Autodesk Fusion 360 part; units mm, degrees
(part 2 of 2)
sketch "Sketch23" plane through (0, 5, 0) normal (0, 1, 0) x (-1, 0, 0)
  circle A0 centre (-181.5, -92.25) radius 5
  circle A1 centre (-181.5, -115.25) radius 5
  circle A2 centre (-154.5, -126.75) radius 5
  circle A3 centre (-154.5, -103.75) radius 5
  circle A4 centre (-186.75, -72.25) radius 4
  circle A5 centre (-140.75, -72.25) radius 4
  circle A6 centre (-94.75, -72.25) radius 4
  circle A7 centre (-48.75, -72.25) radius 4
  circle A8 centre (-190, -170) radius 3.75
  circle A9 centre (-13.25, -72.25) radius 4
  circle A10 centre (-59.25, -72.25) radius 4
  circle A11 centre (-105.25, -72.25) radius 4
  circle A12 centre (-151.25, -72.25) radius 4
  circle A13 centre (-154.5, -92.25) radius 5
  circle A14 centre (-154.5, -115.25) radius 5
  circle A15 centre (-181.5, -126.75) radius 5
  circle A16 centre (-181.5, -103.75) radius 5
  line L0 (-116.5, -98) -> (-126.5, -98)
  line L1 (-126.5, -98) -> (-126.5, -88)
  line L2 (-126.5, -88) -> (-116.5, -88)
  line L3 (-116.5, -88) -> (-116.5, -98)
  line L4 (0, -101) -> (-8, -101)
  line L5 (-8, -101) -> (-8, -85)
  line L6 (-8, -85) -> (0, -85)
  line L7 (0, -85) -> (0, -67)
  line L8 (0, -67) -> (-8, -67)
  line L9 (-8, -67) -> (-8, -51)
  line L10 (-8, -51) -> (0, -51)
  line L11 (0, -51) -> (0, -11)
  line L12 (0, -11) -> (-6.3858, -11)
  arc A17 (-12.9938, -7.7418) -> (-6.3858, -11) centre (-10, -10) ccw
  arc A18 (-14.6419, 0) -> (-12.9938, -7.7418) centre (-13.25, -3.75) ccw
  line L13 (-14.6419, 0) -> (-47.3581, 0)
  arc A19 (-50.1419, 0) -> (-47.3581, 0) centre (-48.75, -3.75) ccw
  line L14 (-50.1419, 0) -> (-57.8581, 0)
  arc A20 (-60.6419, 0) -> (-57.8581, 0) centre (-59.25, -3.75) ccw
  line L15 (-60.6419, 0) -> (-93.3581, 0)
  arc A21 (-96.1419, 0) -> (-93.3581, 0) centre (-94.75, -3.75) ccw
  line L16 (-96.1419, 0) -> (-103.8581, 0)
  arc A22 (-106.6419, 0) -> (-103.8581, 0) centre (-105.25, -3.75) ccw
  line L17 (-106.6419, 0) -> (-139.3581, 0)
  arc A23 (-142.1419, 0) -> (-139.3581, 0) centre (-140.75, -3.75) ccw
  line L18 (-142.1419, 0) -> (-149.8581, 0)
  arc A24 (-152.6419, 0) -> (-149.8581, 0) centre (-151.25, -3.75) ccw
  line L19 (-152.6419, 0) -> (-185.3581, 0)
  arc A25 (-187.0062, -7.7418) -> (-185.3581, 0) centre (-186.75, -3.75) ccw
  arc A26 (-193.6142, -11) -> (-187.0062, -7.7418) centre (-190, -10) ccw
  line L20 (-193.6142, -11) -> (-200, -11)
  line L21 (-200, -11) -> (-200, -65)
  line L22 (-200, -65) -> (-192, -65)
  line L23 (-192, -65) -> (-192, -78)
  line L24 (-192, -78) -> (-200, -78)
  line L25 (-200, -78) -> (-200, -180)
  line L26 (-200, -180) -> (-180, -180)
  line L27 (-180, -180) -> (-180, -140)
  line L28 (-180, -140) -> (-124.5, -140)
  line L29 (-124.5, -140) -> (-124.5, -110)
  line L30 (-124.5, -110) -> (-55.5, -110)
  line L31 (-55.5, -110) -> (-55.5, -140)
  line L32 (-55.5, -140) -> (-8, -140)
  line L33 (-8, -140) -> (-8, -129)
  line L34 (-8, -129) -> (0, -129)
  line L35 (0, -129) -> (0, -101)
  line L36 (-55.5, -110) -> (-124.5, -110)
  line L37 (-124.5, -110) -> (-124.5, -115)
  line L38 (-124.5, -115) -> (-55.5, -115)
  line L39 (-55.5, -115) -> (-55.5, -110)
  dimension "d326" = 69
  dimension "d327" = 5
  constraint horizontal L36
  constraint vertical L37
  constraint horizontal L38
  constraint vertical L39
  constraint coincident L30.end L31.start
  measures "d326" distance of L30.end L29.end
  measures "d327" distance of L30.end L38.end
extrude "Extrude18" add sketch "Sketch23" along normal blind 11.5 separate body contours L29 L30 L31 L36 L37 L38 L39 makes body 3
combine "Combine1" operation cut target body 3 tool bodies 1 keep tools
sketch "Sketch24" plane through (0, 16.5, 0) normal (0, 1, 0) x (-1, 0, 0)
  line L0 (-119.5, -110) -> (-119.5, -115)
  line L1 (-119.5, -115) -> (-60.5, -115)
  line L2 (-60.5, -115) -> (-60.5, -110)
  line L3 (-60.5, -110) -> (-119.5, -110)
  line L4 (-119.5, -115) -> (-115.5, -115)
  line L5 (-115.5, -115) -> (-115.5, -119)
  line L6 (-115.5, -119) -> (-119.5, -119)
  line L7 (-119.5, -119) -> (-119.5, -115)
  dimension "d330" = 4
  dimension "d331" = 4
  constraint horizontal L4
  constraint vertical L5
  constraint horizontal L6
  constraint vertical L7
  constraint coincident L0.end L1.start
  measures "d330" distance of L0.end L4.end
  measures "d331" distance of L0.end L6.end
extrude "Extrude19" add sketch "Sketch24" against normal blind 5 contours L1 L4 L5 L6 L7 bodies 3
hole "Hole35" at (78.25, 10, -112.5) direction (0, -1, 0) diameter 2.5 end through all bodies 1
hole "Hole36" at (101.75, 10, -112.5) direction (0, -1, 0) diameter 2.5 end through all bodies 1
sketch "Sketch26" plane through (0, 10, 0) normal (0, 1, 0) x (-1, 0, 0)
  circle A0 centre (-78.25, -112.5) radius 1.25
  line L0 (-68.5, -115) -> (-68.5, -110)
  line L1 (-68.5, -110) -> (-88, -110)
  line L2 (-88, -110) -> (-88, -115)
  line L3 (-88, -115) -> (-68.5, -115)
  circle A1 centre (-78.25, -112.5) radius 1.5
  dimension "d341" = 3
  constraint concentric A0 A1
  measures "d341" diameter of A1
extrude "Extrude20" cut sketch "Sketch26" along normal up to surface (6.5 mm away) contours A0 | A1 bodies 3
sketch "Sketch27" plane through (0, 10, 0) normal (0, 1, 0) x (-1, 0, 0)
  circle A0 centre (-101.75, -112.5) radius 1.25
  line L0 (-92, -115) -> (-92, -110)
  line L1 (-92, -110) -> (-111.5, -110)
  line L2 (-111.5, -110) -> (-111.5, -115)
  line L3 (-111.5, -115) -> (-92, -115)
  circle A1 centre (-101.75, -112.5) radius 1.5
  dimension "d344" = 3
  constraint concentric A0 A1
  measures "d344" diameter of A1
extrude "Extrude21" cut sketch "Sketch27" along normal up to surface (6.5 mm away) contours A0 | A1 bodies 3
extrude "Extrude22" cut 1 faces at (60.5, 12.1667, -113.3333) along direction (1, 0, 0) blind 0.5 on bodies 3 bodies 3
extrude "Extrude23" cut 1 faces at (64.5, 9, -111.6667) along direction (1, 0, 0) blind 0.5 on bodies 3 bodies 3
extrude "Extrude24" cut 1 faces at (68.5, 9, -111.6667) along direction (-1, 0, 0) blind 0.5 on bodies 3 bodies 3
extrude "Extrude25" cut 1 faces at (88, 8, -111.6667) along direction (1, 0, 0) blind 0.5 on bodies 3 bodies 3
extrude "Extrude26" cut 1 faces at (92, 9, -111.6667) along direction (-1, 0, 0) blind 0.5 on bodies 3 bodies 3
extrude "Extrude27" cut 1 faces at (111.5, 9, -111.6667) along direction (1, 0, 0) blind 0.5 on bodies 3 bodies 3
extrude "Extrude28" cut 1 faces at (119.5, 11.6667, -111.6667) along direction (-1, 0, 0) blind 0.5 on bodies 3 bodies 3
extrude "Extrude29" cut 1 faces at (115.5, 14.8333, -116.3333) along direction (1, 0, 0) blind 0.5 on bodies 3 bodies 3
extrude "Extrude30" cut 1 faces at (117, 14.8333, -119) along direction (0, 0, 1) blind 0.5 on bodies 3 bodies 3
sketch "Sketch28" plane through (0, 75, 0) normal (0, 1, 0) x (-1, 0, 0)
  line L0 (-180, -145) -> (-5, -145)
  line L1 (-5, -145) -> (-5, -175)
  line L2 (-5, -175) -> (-180, -175)
  line L3 (-180, -175) -> (-180, -180)
  line L4 (-180, -180) -> (0, -180)
  line L5 (0, -180) -> (0, -140)
  line L6 (0, -140) -> (-180, -140)
  line L7 (-180, -140) -> (-180, -145)
  line L8 (0, -180) -> (-180, -180)
  line L9 (-180, -180) -> (-180, -140)
  line L10 (-180, -140) -> (0, -140)
  line L11 (0, -140) -> (0, -180)
  line L12 (-185.5, -134.5) -> (5.5, -134.5)
  line L13 (5.5, -134.5) -> (5.5, -185.5)
  line L14 (5.5, -185.5) -> (-185.5, -185.5)
  line L15 (-185.5, -185.5) -> (-185.5, -134.5)
  line L16 (-180.5, -139.5) -> (0.5, -139.5)
  line L17 (0.5, -139.5) -> (0.5, -180.5)
  line L18 (0.5, -180.5) -> (-180.5, -180.5)
  line L19 (-180.5, -180.5) -> (-180.5, -139.5)
  constraint horizontal L8
  constraint vertical L9
  constraint horizontal L10
  constraint vertical L11
  constraint coincident L6.end L7.start
  constraint coincident L4.end L5.start
extrude "Extrude33" add sketch "Sketch28" against normal blind 15 separate body contours L12 L13 L14 L15 makes body 4
extrude "Extrude34" add sketch "Sketch28" along normal blind 5 contours L0 L1 L2 L3 L4 L5 L6 L7 L8 L9 L10 L11 | L0 L1 L2 L9 | L12 L13 L14 L15 | L16 L17 L18 L19 bodies 4
sketch "Sketch29" plane through (0, 0, -140) normal (0, 0, 1) x (1, 0, 0)
  arc A0 (6, 7) -> (8, 5) centre (8, 7) ccw
  line L0 (8, 5) -> (55.5, 5)
  line L1 (55.5, 5) -> (55.5, 16.5)
  line L2 (55.5, 16.5) -> (118.5, 16.5)
  line L3 (118.5, 16.5) -> (118.5, 35)
  line L4 (118.5, 35) -> (124.5, 35)
  line L5 (124.5, 35) -> (124.5, 5)
  line L6 (124.5, 5) -> (180, 5)
  line L7 (180, 5) -> (180, 75)
  line L8 (180, 75) -> (0, 75)
  line L9 (0, 75) -> (0, 35)
  line L10 (0, 35) -> (6, 35)
  line L11 (6, 35) -> (6, 7)
  line L12 (180, 75) -> (170, 75)
  line L13 (170, 75) -> (170, 70)
  line L14 (170, 70) -> (180, 70)
  line L15 (180, 70) -> (180, 75)
  line L16 (170, 70) -> (165, 70)
  line L17 (165, 70) -> (165, 65)
  line L18 (165, 65) -> (170, 65)
  line L19 (170, 65) -> (170, 70)
  line L20 (0, 75) -> (10, 75)
  line L21 (10, 75) -> (10, 70)
  line L22 (10, 70) -> (0, 70)
  line L23 (0, 70) -> (0, 75)
  line L24 (10, 70) -> (15, 70)
  line L25 (15, 70) -> (15, 65)
  line L26 (15, 65) -> (10, 65)
  line L27 (10, 65) -> (10, 70)
  line L28 (165, 65) -> (170, 70)
  line L29 (15, 70) -> (10, 65)
  circle A1 centre (12.5, 67.5) radius 1.25
  circle A2 centre (167.5, 67.5) radius 1.25
  circle A3 centre (12.5, 67.5) radius 1.75
  circle A4 centre (167.5, 67.5) radius 1.75
  dimension "d377" = 10
  dimension "d378" = 5
  dimension "d379" = 5
  dimension "d380" = 5
  dimension "d381" = 10
  dimension "d382" = 5
  dimension "d383" = 5
  dimension "d384" = 5
  dimension "d385" = 2.5
  dimension "d386" = 2.5
  dimension "d399" = 3.5
  dimension "d400" = 3.5
  constraint horizontal L12
  constraint vertical L13
  constraint horizontal L14
  constraint vertical L15
  constraint coincident L7.end L8.start
  constraint horizontal L16
  constraint vertical L17
  constraint horizontal L18
  constraint vertical L19
  constraint horizontal L20
  constraint vertical L21
  constraint horizontal L22
  constraint vertical L23
  constraint coincident L8.end L9.start
  constraint horizontal L24
  constraint vertical L25
  constraint horizontal L26
  constraint vertical L27
  constraint midpoint L29 A1.centre
  constraint midpoint L28 A2.centre
  constraint concentric A1 A3
  constraint concentric A2 A4
  measures "d377" distance of L7.end L12.end
  measures "d378" distance of L7.end L14.end
  measures "d379" distance of L13.end L16.end
  measures "d380" distance of L13.end L18.end
  measures "d381" distance of L8.end L20.end
  measures "d382" distance of L8.end L22.end
  measures "d383" distance of L21.end L24.end
  measures "d384" distance of L21.end L26.end
  measures "d385" diameter of A1
  measures "d386" diameter of A2
  measures "d399" diameter of A3
  measures "d400" diameter of A4
extrude "Extrude35" cut sketch "Sketch29" against normal up to surface (5 mm away) contours L29 A1 | L29 A1 | L28 A2 | L28 A2 bodies 1
sketch "Sketch30" plane through (0, 0, 0) normal (-1, 0, 0) x (0, 0, 1)
  line L0 (-180, 0) -> (0, 0)
  line L1 (0, 0) -> (0, 35)
  line L2 (0, 35) -> (-6, 35)
  line L3 (-6, 35) -> (-6, 10)
  arc A0 (-11, 5) -> (-6, 10) centre (-11, 10) ccw
  line L4 (-11, 5) -> (-51, 5)
  arc A1 (-56, 10) -> (-51, 5) centre (-51, 10) ccw
  line L5 (-56, 10) -> (-56, 35)
  line L6 (-56, 35) -> (-62, 35)
  line L7 (-62, 35) -> (-62, 10)
  arc A2 (-67, 5) -> (-62, 10) centre (-67, 10) ccw
  line L8 (-67, 5) -> (-85, 5)
  arc A3 (-90, 10) -> (-85, 5) centre (-85, 10) ccw
  line L9 (-90, 10) -> (-90, 35)
  line L10 (-90, 35) -> (-96, 35)
  line L11 (-96, 35) -> (-96, 10)
  arc A4 (-101, 5) -> (-96, 10) centre (-101, 10) ccw
  line L12 (-101, 5) -> (-129, 5)
  arc A5 (-134, 10) -> (-129, 5) centre (-129, 10) ccw
  line L13 (-134, 10) -> (-134, 35)
  line L14 (-134, 35) -> (-140, 35)
  line L15 (-140, 35) -> (-140, 75)
  line L16 (-140, 75) -> (-180, 75)
  line L17 (-180, 75) -> (-180, 0)
  line L18 (-180, 75) -> (-140, 75)
  line L19 (-140, 75) -> (-140, 70)
  line L20 (-140, 70) -> (-180, 70)
  line L21 (-180, 70) -> (-180, 75)
  line L22 (-160, 75) -> (-160, 70)
  line L23 (-160, 70) -> (-162.5, 70)
  line L24 (-162.5, 70) -> (-162.5, 65)
  line L25 (-162.5, 65) -> (-160, 65)
  line L26 (-160, 65) -> (-160, 70)
  line L27 (-160, 70) -> (-157.5, 70)
  line L28 (-157.5, 70) -> (-157.5, 65)
  line L29 (-157.5, 65) -> (-160, 65)
  line L30 (-160, 65) -> (-160, 70)
  circle A6 centre (-160, 67.5) radius 1.25
  circle A7 centre (-160, 67.5) radius 1.75
  dimension "d389" = 40
  dimension "d390" = 5
  dimension "d391" = 2.5
  dimension "d392" = 5
  dimension "d393" = 2.5
  dimension "d394" = 5
  dimension "d395" = 2.5
  dimension "d401" = 3.5
  constraint horizontal L18
  constraint vertical L19
  constraint horizontal L20
  constraint vertical L21
  constraint coincident L16.end L17.start
  constraint midpoint L18 L22.start
  constraint midpoint L20 L22.end
  constraint horizontal L23
  constraint vertical L24
  constraint horizontal L25
  constraint vertical L26
  constraint horizontal L27
  constraint vertical L28
  constraint horizontal L29
  constraint vertical L30
  constraint midpoint L26 A6.centre
  constraint concentric A6 A7
  measures "d389" distance of L16.end L15.end
  measures "d390" distance of L16.end L20.end
  measures "d391" distance of L22.end L23.end
  measures "d392" distance of L22.end L25.end
  measures "d393" distance of L22.end L27.end
  measures "d394" distance of L22.end L25.end
  measures "d395" diameter of A6
  measures "d401" diameter of A7
extrude "Extrude36" cut sketch "Sketch30" against normal up to surface (5 mm away) contours L26 L30 A6 | L26 L30 A6 bodies 1
extrude "Extrude37" cut sketch "Sketch29" along normal up to surface (5.5 mm away) contours L29 A1 A3 | L29 A1 A3 | L29 A1 | L29 A1 | L28 A2 A4 | L28 A2 A4 | L28 A2 | L28 A2 bodies 4
extrude "Extrude38" cut sketch "Sketch30" along normal up to surface (5.5 mm away) contours L26 L30 A6 A7 | L26 L30 A6 A7 | L26 L30 A6 | L26 L30 A6 bodies 4
sketch "Sketch31" plane through (185.5, 0, 0) normal (1, 0, 0) x (0, 0, -1)
  line L0 (134.5, 80) -> (134.5, 60)
  line L1 (134.5, 60) -> (185.5, 60)
  line L2 (185.5, 60) -> (185.5, 80)
  line L3 (185.5, 80) -> (134.5, 80)
  line L4 (134.5, 80) -> (185.5, 80)
  line L5 (185.5, 80) -> (185.5, 75)
  line L6 (185.5, 75) -> (134.5, 75)
  line L7 (134.5, 75) -> (134.5, 80)
  line L8 (134.5, 75) -> (140, 75)
  line L9 (140, 75) -> (140, 60)
  line L10 (140, 60) -> (134.5, 60)
  line L11 (134.5, 60) -> (134.5, 75)
  line L12 (185.5, 75) -> (180, 75)
  line L13 (180, 75) -> (180, 60)
  line L14 (180, 60) -> (185.5, 60)
  line L15 (185.5, 60) -> (185.5, 75)
  line L16 (140, 75) -> (145, 75)
  line L17 (145, 75) -> (145, 60)
  line L18 (145, 60) -> (140, 60)
  line L19 (140, 60) -> (140, 75)
  line L20 (180, 75) -> (175, 75)
  line L21 (175, 75) -> (175, 60)
  line L22 (175, 60) -> (180, 60)
  line L23 (180, 60) -> (180, 75)
  dimension "d406" = 5
  dimension "d407" = 5.5
  dimension "d408" = 5.5
  dimension "d409" = 5
  dimension "d410" = 5
  constraint horizontal L4
  constraint vertical L5
  constraint horizontal L6
  constraint vertical L7
  constraint coincident L0.start L3.end
  constraint collinear L2 L5
  constraint horizontal L8
  constraint vertical L9
  constraint horizontal L10
  constraint vertical L11
  constraint collinear L1 L10
  constraint horizontal L12
  constraint vertical L13
  constraint horizontal L14
  constraint vertical L15
  constraint collinear L1 L14
  constraint horizontal L16
  constraint vertical L17
  constraint horizontal L18
  constraint vertical L19
  constraint horizontal L20
  constraint vertical L21
  constraint horizontal L22
  constraint vertical L23
  constraint collinear L1 L18
  constraint collinear L1 L22
  measures "d406" distance of L0.start L6.end
  measures "d407" distance of L6.end L8.end
  measures "d408" distance of L5.end L12.end
  measures "d409" distance of L8.end L16.end
  measures "d410" distance of L12.end L20.end
extrude "Extrude39" cut sketch "Sketch31" against normal up to surface (5 mm away) contours L1 L6 L17 L21 bodies 4
sketch "Sketch32" plane through (0, 40, 0) normal (0, 1, 0) x (-1, 0, 0)
  circle A0 centre (-3, -3) radius 1.75
  circle A1 centre (-121.5, -137) radius 1.75
  circle A2 centre (-121.5, -93) radius 1.75
  circle A3 centre (-197, -3) radius 1.75
  circle A4 centre (-3, -59) radius 1.75
  circle A5 centre (-3, -137) radius 1.75
  circle A6 centre (-3, -93) radius 1.75
  circle A7 centre (-197, -73) radius 1.75
  line L0 (-124.5, -140) -> (0, -140)
  line L1 (0, -140) -> (0, 0)
  line L2 (0, 0) -> (-200, 0)
  line L3 (-200, 0) -> (-200, -76)
  line L4 (-200, -76) -> (-124.5, -76)
  line L5 (-124.5, -76) -> (-124.5, -140)
  line L6 (-100, 0) -> (-100, -140)
  circle A8 centre (-100, 0) radius 10
  circle A9 centre (-100, -35) radius 10
  circle A10 centre (-100, -70) radius 10
  circle A11 centre (-100, -105) radius 10
  circle A12 centre (-100, -140) radius 10
  line L7 (-21.5, -113) -> (-78.5, -113)
  line L8 (-78.5, -113) -> (-78.5, 0)
  line L9 (-78.5, 0) -> (-21.5, 0)
  line L10 (-21.5, 0) -> (-21.5, -113)
  line L11 (-21.5, -113) -> (-78.5, 0) construction
  line L12 (-78.5, -113) -> (-21.5, 0) construction
  line L13 (-25.5, -4) -> (-25.5, -109)
  line L14 (-25.5, -109) -> (-74.5, -109)
  line L15 (-74.5, -109) -> (-74.5, -4)
  line L16 (-74.5, -4) -> (-25.5, -4)
  circle A13 centre (-74.5, -109) radius 3
  circle A14 centre (-25.5, -109) radius 3
  line L17 (-78.5, 0) -> (-69.25, 0)
  line L18 (-69.25, 0) -> (-69.25, -113)
  line L19 (-69.25, -113) -> (-78.5, -113)
  line L20 (-78.5, -113) -> (-78.5, 0)
  line L21 (-21.5, 0) -> (-30.75, 0)
  line L22 (-30.75, 0) -> (-30.75, -113)
  line L23 (-30.75, -113) -> (-21.5, -113)
  line L24 (-21.5, -113) -> (-21.5, 0)
  line L25 (-78.5, -113) -> (-21.5, -113)
  line L26 (-21.5, -113) -> (-21.5, -46.5)
  line L27 (-21.5, -46.5) -> (-78.5, -46.5)
  line L28 (-78.5, -46.5) -> (-78.5, -113)
  circle A15 centre (-30.75, -46.5) radius 3
  circle A16 centre (-69.25, -46.5) radius 3
  line L29 (-78.5, 0) -> (-21.5, 0)
  line L30 (-21.5, 0) -> (-21.5, -13.75)
  line L31 (-21.5, -13.75) -> (-78.5, -13.75)
  line L32 (-78.5, -13.75) -> (-78.5, 0)
  line L33 (-78.5, 0) -> (-74.5, 0)
  line L34 (-74.5, 0) -> (-74.5, -6)
  line L35 (-74.5, -6) -> (-78.5, -6)
  line L36 (-78.5, -6) -> (-78.5, 0)
  line L37 (-21.5, -13.75) -> (-25.5, -13.75)
  line L38 (-25.5, -13.75) -> (-25.5, -19.75)
  line L39 (-25.5, -19.75) -> (-21.5, -19.75)
  line L40 (-21.5, -19.75) -> (-21.5, -13.75)
  line L41 (-74.5, 0) -> (-72.5, 0)
  line L42 (-72.5, 0) -> (-72.5, -4)
  line L43 (-72.5, -4) -> (-74.5, -4)
  line L44 (-74.5, -4) -> (-74.5, 0)
  point P0 (-50, -56.5)
  dimension "d415" = 20
  dimension "d418" = 140
  dimension "d419" = 0
  dimension "d420" = 57
  dimension "d421" = 113
  dimension "d422" = 4
  dimension "d423" = 6
  dimension "d424" = 6
  dimension "d425" = 9.25
  dimension "d426" = 9.25
  dimension "d427" = 66.5
  dimension "d428" = 6
  dimension "d429" = 6
  dimension "d430" = 57
  dimension "d431" = 13.75
  dimension "d432" = 4
  dimension "d433" = 6
  dimension "d434" = 4
  dimension "d435" = 6
  dimension "d440" = 2
  dimension "d441" = 4
  constraint midpoint L2 L6.start
  constraint coincident L0 L6.end
  constraint perpendicular L0 L6
  constraint coincident L6.start A8.centre
  constraint horizontal L7
  constraint perpendicular L7 L8
  constraint parallel L7 L9
  constraint parallel L8 L10
  constraint coincident L11 P0
  constraint coincident L12 P0
  constraint coincident L14.end L15.start
  constraint coincident L13.end L14.start
  constraint horizontal L17
  constraint vertical L18
  constraint horizontal L19
  constraint vertical L20
  constraint horizontal L21
  constraint vertical L22
  constraint horizontal L23
  constraint vertical L24
  constraint collinear L7 L23
  constraint collinear L7 L19
  constraint horizontal L25
  constraint vertical L26
  constraint horizontal L27
  constraint vertical L28
  constraint coincident L22 A15.centre
  constraint coincident L27 A15.centre
  constraint coincident L27 A16.centre
  constraint coincident L18 A16.centre
  constraint coincident L7.start L26
  constraint horizontal L29
  constraint vertical L30
  constraint horizontal L31
  constraint vertical L32
  constraint horizontal L33
  constraint vertical L34
  constraint horizontal L35
  constraint vertical L36
  constraint horizontal L37
  constraint vertical L38
  constraint horizontal L39
  constraint vertical L40
  constraint horizontal L41
  constraint vertical L42
  constraint horizontal L43
  constraint vertical L44
  constraint collinear L2 L29
  measures "d415" diameter of A8
  measures "d420" distance of L8.end L9.end
  measures "d421" distance of L7.end L8.end
  measures "d423" diameter of A13
  measures "d424" diameter of A14
  measures "d425" distance of L8.end L17.end
  measures "d426" distance of L9.end L21.end
  measures "d427" distance of L7.end L27.end
  measures "d428" diameter of A15
  measures "d429" diameter of A16
  measures "d430" distance of L8.end L9.end
  measures "d431" distance of L8.end L31.end
  measures "d432" distance of L8.end L33.end
  measures "d433" distance of L8.end L35.end
  measures "d434" distance of L30.end L37.end
  measures "d435" distance of L30.end L39.end
  measures "d440" distance of L33.end L41.end
  measures "d441" distance of L33.end L15.end
extrude "Extrude40" add sketch "Sketch32" along normal blind 5 contours L10 L13 L24 L31 L37 L38 L39 L40 | L2 L9 L16 L17 L29 L34 L41 L42 L43 L44 | L2 L8 L9 L15 L17 L20 L29 L32 L33 L34 L35 L36 L44 | L22 L27 A15 | L22 L27 A15 | L18 L27 A16 | L18 L27 A16 | L22 L27 A15 | L22 L27 A15 | L13 L14 A14 | L13 L14 A14 | L18 L27 A16 | L18 L27 A16 | L14 L15 A13 | L14 L15 A13 bodies 2
extrude "Extrude41" add 2 faces at (22.8333, 45, -17.75) (77.1667, 45, -3.3333) along direction (0, 1, 0) blind 1 on bodies 2 bodies 2
hole "Hole37" at (69.25, 45, -46.5) direction (0, -1, 0) diameter 2.5 end up to surface (10 mm away) bodies 2
hole "Hole38" at (30.75, 45, -46.5) direction (0, -1, 0) diameter 2.5 end up to surface (10 mm away) bodies 2
hole "Hole39" at (74.5, 45, -109) direction (0, -1, 0) diameter 2.5 end up to surface (10 mm away) bodies 2
hole "Hole40" at (25.5, 45, -109) direction (0, -1, 0) diameter 2.5 end up to surface (10 mm away) bodies 2
fillet "Fillet5" radius 2 8 edges at (28.297, 40, -107.9152) (77.297, 40, -107.9152) (33.547, 40, -45.4152) (72.047, 40, -45.4152) (23.5, 40, -13.75) (21.5, 40, -16.75) (25.5, 40, -16.75) (23.5, 40, -19.75) on bodies 2
fillet "Fillet5" radius 2 3 edges at (78.5, 40, -3) (76.5, 40, -6) (72.5, 40, -2) on bodies 2
fillet "Fillet6" radius 2 2 edges at (74.5, 40, -5) (73.5, 40, -4) on bodies 2
extrude "Extrude42" cut sketch "Sketch32" against normal up to surface (5 mm away) contours L6 A11 | L6 A11 | L6 A10 | L6 A10 | L6 A9 | L6 A9 bodies 2
sketch "Sketch33" plane through (0, 16.5, 0) normal (0, 1, 0) x (-1, 0, 0)
  circle A0 centre (-101.75, -112.5) radius 1.5
  circle A1 centre (-78.25, -112.5) radius 1.5
  line L0 (-119, -110) -> (-119, -118.5)
  line L1 (-119, -118.5) -> (-116, -118.5)
  line L2 (-116, -118.5) -> (-116, -115)
  line L3 (-61, -115) -> (-61, -110)
  circle A2 centre (-78.25, -112.5) radius 3.25
  circle A3 centre (-101.75, -112.5) radius 3.25
  line L4 (-61, -110) -> (-119, -110)
  line L5 (-116, -115) -> (-61, -115)
  point P0 (-78.25, -112.5)
  point P1 (-101.75, -112.5)
  dimension "d468" = 6.5
  dimension "d469" = 6.5
  constraint coincident P0 A1.centre
  constraint coincident A0.centre A3.centre
  constraint coincident P1 A0.centre
  measures "d468" diameter of A2
  measures "d469" diameter of A3
extrude "Extrude43" cut sketch "Sketch33" against normal blind 2.5 contours A3 L4 L5 | A3 L4 | A3 L5 | A2 L4 L5 | A2 L4 | A2 L5 bodies 3
sketch "Sketch34" plane through (0, 0, -134.5) normal (0, 0, 1) x (1, 0, 0)
  circle A0 centre (167.5, 67.5) radius 1.75
  circle A1 centre (12.5, 67.5) radius 1.75
  line L0 (-5.5, 80) -> (-5.5, 60)
  line L1 (-5.5, 60) -> (185.5, 60)
  line L2 (185.5, 60) -> (185.5, 80)
  line L3 (185.5, 80) -> (-5.5, 80)
  circle A2 centre (12.5, 67.5) radius 3.25
  circle A3 centre (167.5, 67.5) radius 3.25
  dimension "d470" = 6.5
  dimension "d471" = 6.5
  constraint concentric A1 A2
  constraint concentric A0 A3
  measures "d470" diameter of A2
  measures "d471" diameter of A3
extrude "Extrude44" cut sketch "Sketch34" against normal blind 2.5 contours A2 | A3 bodies 4
sketch "Sketch35" plane through (-5.5, 0, 0) normal (-1, 0, 0) x (0, 0, 1)
  circle A0 centre (-160, 67.5) radius 1.75
  line L0 (-185.5, 80) -> (-185.5, 60)
  line L1 (-185.5, 60) -> (-134.5, 60)
  line L2 (-134.5, 60) -> (-134.5, 80)
  line L3 (-134.5, 80) -> (-185.5, 80)
  circle A1 centre (-160, 67.5) radius 3.25
  dimension "d474" = 6.5
  constraint concentric A0 A1
  measures "d474" diameter of A1
extrude "Extrude45" cut sketch "Sketch35" against normal blind 2.5 contours A1 bodies 4
sketch "Sketch36" plane through (0, 40, 0) normal (0, 1, 0) x (-1, 0, 0)
  circle A0 centre (-100, -105) radius 10
  circle A1 centre (-100, -70) radius 10
  circle A2 centre (-100, -35) radius 10
  circle A3 centre (-74.5, -109) radius 5
  circle A4 centre (-30.75, -46.5) radius 5
  circle A5 centre (-3, -3) radius 1.75
  circle A6 centre (-121.5, -137) radius 1.75
  circle A7 centre (-121.5, -93) radius 1.75
  circle A8 centre (-197, -3) radius 1.75
  circle A9 centre (-3, -59) radius 1.75
  circle A10 centre (-3, -137) radius 1.75
  circle A11 centre (-3, -93) radius 1.75
  circle A12 centre (-197, -73) radius 1.75
  line L0 (-124.5, -140) -> (0, -140)
  line L1 (0, -140) -> (0, 0)
  line L2 (-80.5, 0) -> (-200, 0)
  line L3 (-200, 0) -> (-200, -76)
  line L4 (-200, -76) -> (-124.5, -76)
  line L5 (-124.5, -76) -> (-124.5, -140)
  line L6 (-19.5, -21.75) -> (-27.5, -21.75)
  line L7 (-27.5, -21.75) -> (-27.5, -11.75)
  line L8 (-27.5, -11.75) -> (-19.5, -11.75)
  line L9 (-19.5, -11.75) -> (-19.5, -21.75)
  circle A13 centre (-25.5, -109) radius 5
  circle A14 centre (-69.25, -46.5) radius 5
  line L10 (0.25, -140.25) -> (-6.25, -140.25)
  line L11 (-6.25, -140.25) -> (-6.25, -133.75)
  line L12 (-6.25, -133.75) -> (0.25, -133.75)
  line L13 (0.25, -133.75) -> (0.25, -140.25)
  line L14 (0.25, -140.25) -> (-6.25, -133.75) construction
  line L15 (-6.25, -140.25) -> (0.25, -133.75) construction
  line L16 (0.25, -6.25) -> (-6.25, -6.25)
  line L17 (-6.25, -6.25) -> (-6.25, 0.25)
  line L18 (-6.25, 0.25) -> (0.25, 0.25)
  line L19 (0.25, 0.25) -> (0.25, -6.25)
  line L20 (0.25, -6.25) -> (-6.25, 0.25) construction
  line L21 (-6.25, -6.25) -> (0.25, 0.25) construction
  line L22 (-200.25, -6.25) -> (-193.75, -6.25)
  line L23 (-193.75, -6.25) -> (-193.75, 0.25)
  line L24 (-193.75, 0.25) -> (-200.25, 0.25)
  line L25 (-200.25, 0.25) -> (-200.25, -6.25)
  line L26 (-200.25, -6.25) -> (-193.75, 0.25) construction
  line L27 (-193.75, -6.25) -> (-200.25, 0.25) construction
  line L28 (-200.25, -76.25) -> (-193.75, -76.25)
  line L29 (-193.75, -76.25) -> (-193.75, -69.75)
  line L30 (-193.75, -69.75) -> (-200.25, -69.75)
  line L31 (-200.25, -69.75) -> (-200.25, -76.25)
  line L32 (-200.25, -76.25) -> (-193.75, -69.75) construction
  line L33 (-193.75, -76.25) -> (-200.25, -69.75) construction
  line L34 (-118.25, -140.25) -> (-124.75, -140.25)
  line L35 (-124.75, -140.25) -> (-124.75, -133.75)
  line L36 (-124.75, -133.75) -> (-118.25, -133.75)
  line L37 (-118.25, -133.75) -> (-118.25, -140.25)
  line L38 (-118.25, -140.25) -> (-124.75, -133.75) construction
  line L39 (-124.75, -140.25) -> (-118.25, -133.75) construction
  circle A15 centre (-121.5, -93) radius 3.25
  circle A16 centre (-3, -93) radius 3.25
  circle A17 centre (-3, -59) radius 3.25
  line L40 (-70.5, 0) -> (-70.5, -6)
  line L41 (-70.5, -6) -> (-72.5, -6)
  line L42 (-72.5, -6) -> (-72.5, -8)
  line L43 (-72.5, -8) -> (-80.5, -8)
  line L44 (-80.5, -8) -> (-80.5, 0)
  line L45 (0, 0) -> (-70.5, 0)
  point P0 (-3, -137)
  point P1 (-3, -3)
  point P2 (-197, -3)
  point P3 (-197, -73)
  point P4 (-121.5, -137)
  dimension "d477" = 6.5
  dimension "d478" = 6.5
  dimension "d479" = 6.5
  dimension "d480" = 6.5
  dimension "d481" = 6.5
  dimension "d482" = 6.5
  dimension "d483" = 6.5
  dimension "d484" = 6.5
  dimension "d485" = 6.5
  dimension "d486" = 6.5
  dimension "d487" = 6.5
  dimension "d488" = 6.5
  dimension "d489" = 6.5
  constraint horizontal L10
  constraint perpendicular L10 L11
  constraint parallel L10 L12
  constraint parallel L11 L13
  constraint coincident L14 P0
  constraint coincident L15 P0
  constraint coincident P0 A10.centre
  constraint horizontal L16
  constraint perpendicular L16 L17
  constraint parallel L16 L18
  constraint parallel L17 L19
  constraint coincident L20 P1
  constraint coincident L21 P1
  constraint coincident P1 A5.centre
  constraint horizontal L22
  constraint perpendicular L22 L23
  constraint parallel L22 L24
  constraint parallel L23 L25
  constraint coincident L26 P2
  constraint coincident L27 P2
  constraint coincident P2 A8.centre
  constraint horizontal L28
  constraint perpendicular L28 L29
  constraint parallel L28 L30
  constraint parallel L29 L31
  constraint coincident L32 P3
  constraint coincident L33 P3
  constraint coincident P3 A12.centre
  constraint horizontal L34
  constraint perpendicular L34 L35
  constraint parallel L34 L36
  constraint parallel L35 L37
  constraint coincident L38 P4
  constraint coincident L39 P4
  constraint coincident P4 A6.centre
  constraint concentric A7 A15
  constraint concentric A11 A16
  constraint concentric A9 A17
  measures "d477" distance of L11.end L12.end
  measures "d478" distance of L10.end L11.end
  measures "d479" distance of L17.end L18.end
  measures "d480" distance of L16.end L17.end
  measures "d481" distance of L23.end L24.end
  measures "d482" distance of L22.end L23.end
  measures "d483" distance of L29.end L30.end
  measures "d484" distance of L28.end L29.end
  measures "d485" distance of L35.end L36.end
  measures "d486" distance of L34.end L35.end
  measures "d487" diameter of A15
  measures "d488" diameter of A16
  measures "d489" diameter of A17
extrude "Extrude46" cut sketch "Sketch36" against normal blind 2.5 contours L0 L5 L36 L37 | L0 L1 L11 L12 | L5 A15 | L1 A16 | L3 L4 L29 L30 | L1 A17 | L2 L3 L22 L23 | L1 L16 L17 L45 picked at (-124.0833, -93) picked at (-0.4167, -93) picked at (-0.4167, -59) bodies 2
extrude "Extrude47" cut 1 faces at (121.1667, 12.1667, -119) along direction (0, 0, 1) up to surface (9 mm away) on bodies 1 bodies 1
extrude "Extrude48" cut 1 faces at (65, 9, -111.6667) along direction (1, 0, 0) up to surface (54 mm away) on bodies 3 bodies 3
extrude "Extrude49" cut 2 faces at (89.3333, 7, -111.6667) (67.1667, 7, -111.6667) along direction (0, 1, 0) up to surface end surface through (0, 5, 0) normal (0, 1, 0) offset 0 on bodies 1 bodies 1
extrude "Extrude50" cut 1 faces at (68.5, 8.3333, -111.6667) along direction (1, 0, 0) blind 6.5 on bodies 1 bodies 1
extrude "Extrude51" cut 1 faces at (88, 8.3333, -111.6667) along direction (-1, 0, 0) blind 6.5 on bodies 1 bodies 1
extrude "Extrude52" cut 1 faces at (92, 6.6667, -113.3333) along direction (1, 0, 0) blind 6.5 on bodies 1 bodies 1
sketch "Sketch37" plane through (0, 7, 0) normal (0, 1, 0) x (-1, 0, 0)
  line L0 (-115.5, -115) -> (-111.5, -115)
  line L1 (-111.5, -115) -> (-111.5, -110)
  line L2 (-111.5, -110) -> (-119.5, -110)
  line L3 (-119.5, -110) -> (-119.5, -119)
  line L4 (-119.5, -119) -> (-115.5, -119)
  line L5 (-115.5, -119) -> (-115.5, -115)
  line L6 (-111.5, -115) -> (-115.5, -115)
  line L7 (-115.5, -115) -> (-115.5, -110)
  line L8 (-115.5, -110) -> (-111.5, -110)
  line L9 (-111.5, -110) -> (-111.5, -115)
  constraint horizontal L6
  constraint vertical L7
  constraint horizontal L8
  constraint vertical L9
  constraint midpoint L2 L7.end
  constraint coincident L0.end L1.start
extrude "Extrude53" cut sketch "Sketch37" against normal up to surface (2 mm away) contours L0 L1 L2 L6 L7 L8 L9 bodies 1
extrude "Extrude54" cut 1 faces at (111.5, 6.6667, -111.6667) along direction (-1, 0, 0) blind 6.5 on bodies 1 bodies 1
extrude "Extrude55" cut 1 faces at (64.5, 8.3333, -111.6667) along direction (-1, 0, 0) up to surface (3 mm away) on bodies 1 bodies 1
hidden bodies 4
equation "width = 200 mm"
equation "length = 180 mm"
equation "d3 = width"
equation "d4 = length"
equation "height = 5 mm"
equation "d6 = height"
equation "screw_hole_diam = 4 mm"
equation "screw_head_diam = 7.5 mm"
equation "screw_offset = 10 mm"
equation "d12 = -screw_offset"
equation "d19 = ( screw_head_diam - screw_hole_diam ) / 2"
equation "d20 = height"
equation "batt_width = 170 mm"
equation "batt_length = 30 mm"
equation "batt_height = 70 mm"
equation "batt_wall = 5 mm"
equation "d25 = batt_width + batt_wall * 2"
equation "d26 = batt_length + batt_wall * 2"
equation "d27 = batt_wall"
equation "d28 = batt_height"
equation "batt_pwr_height = 10 mm"
equation "batt_cel_length = 4 mm"
equation "d32 = -batt_pwr_height"
equation "d34 = batt_wall"
equation "d35 = batt_cel_length"
equation "batt_cel_height = batt_height - batt_pwr_height - 5 mm"
equation "d37 = -batt_cel_height"
equation "driver_width = 43 mm"
equation "driver_length = 76 mm"
equation "driver_screw_offset = 7.5 mm / 2"
equation "driver_space = 3 mm"
equation "elem_fix_screw_hole_diam = 2 mm + slack_print"
equation "elem_fix_spacer_diam = 6 mm"
equation "elem_fix_spacer_height = 5 mm"
equation "d46 = driver_space / 2"
equation "d47 = driver_length"
equation "d48 = driver_width"
equation "d49 = driver_length"
equation "d50 = driver_space"
equation "d51 = driver_length"
equation "d52 = driver_width"
equation "d53 = driver_length"
equation "d54 = driver_screw_offset"
equation "d55 = driver_screw_offset"
equation "d64 = elem_fix_spacer_height"
equation "d67 = driver_fix_fillet"
equation "elem_fix_fillet = 2 mm"
equation "driver_fix_fillet = 1 mm"
equation "bms_width = 59 mm"
equation "bms_length = 20 mm"
equation "bms_thick = 1.5 mm"
equation "bms_wall = 5 mm"
equation "d78 = ( batt_width + batt_wall * 2 ) / 2 - ( bms_width + bms_wall * 2 ) / 2"
equation "d79 = bms_length + bms_wall * 2"
equation "bms_in_fillet = 1.5 mm"
equation "d81 = bms_width + bms_wall * 2"
equation "d82 = bms_length + bms_wall * 2"
equation "d83 = bms_wall"
equation "d91 = bms_thick + bms_wall * 2"
equation "d93 = bms_wall"
equation "d95 = bms_thick + slack_print"
equation "bms_bottom_slack = 3 mm"
equation "d109 = bms_bottom_slack"
equation "d111 = bms_bottom_slack"
equation "pwr_width = 27 mm"
equation "pwr_interv = 11.5 mm"
equation "pwr_length = pwr_interv * 4 + pwr_interv"
equation "pwr_z_offset = 20 mm"
equation "d121 = driver_length"
equation "pwr_slack = 2.5 mm + 5 mm"
equation "pwr_slack_outside = 5 mm"
equation "d129 = -pwr_slack_outside"
equation "d130 = pwr_slack"
equation "d131 = pwr_width"
equation "d132 = ( pwr_length - pwr_interv * 4 ) / 2"
equation "d133 = pwr_width"
equation "d134 = pwr_interv"
equation "d137 = pwr_width"
equation "d138 = pwr_interv"
equation "pwr_fix_screw_hole_diam = elem_fix_screw_hole_diam"
equation "d148 = elem_fix_spacer_height"
equation "d150 = elem_fix_spacer_height + pwr_z_offset"
equation "d153 = elem_fix_fillet"
equation "d158 = elem_fix_screw_hole_diam"
equation "d161 = elem_fix_screw_hole_diam"
equation "d164 = elem_fix_screw_hole_diam"
equation "d167 = elem_fix_screw_hole_diam"
equation "d170 = elem_fix_screw_hole_diam"
equation "d173 = elem_fix_screw_hole_diam"
equation "d176 = elem_fix_screw_hole_diam"
equation "d179 = elem_fix_screw_hole_diam"
equation "d182 = elem_fix_screw_hole_diam"
equation "d185 = elem_fix_screw_hole_diam"
equation "d188 = elem_fix_screw_hole_diam"
equation "d191 = elem_fix_screw_hole_diam"
equation "d194 = elem_fix_screw_hole_diam"
equation "d197 = elem_fix_screw_hole_diam"
equation "d200 = elem_fix_screw_hole_diam"
equation "d203 = elem_fix_screw_hole_diam"
equation "d206 = pwr_fix_screw_hole_diam"
equation "d209 = pwr_fix_screw_hole_diam"
equation "d212 = pwr_fix_screw_hole_diam"
equation "d215 = pwr_fix_screw_hole_diam"
equation "d217 = height + elem_fix_spacer_height"
equation "d218 = pwr_fix_screw_hole_diam"
equation "d220 = height + elem_fix_spacer_height"
equation "d221 = pwr_fix_screw_hole_diam"
equation "d223 = height + elem_fix_spacer_height"
equation "d224 = pwr_fix_screw_hole_diam"
equation "d226 = height + elem_fix_spacer_height"
equation "d227 = pwr_fix_screw_hole_diam"
equation "floor_spacer_size = 6 mm"
equation "d230 = floor_spacer_size"
equation "d231 = floor_spacer_size"
equation "d232 = floor_spacer_size"
equation "d233 = floor_spacer_size"
equation "d234 = floor_spacer_size"
equation "d235 = floor_spacer_size"
equation "floor_cut_length = length - ( batt_length + batt_wall * 2 ) - driver_length"
equation "d237 = floor_spacer_size"
equation "d238 = floor_cut_length"
equation "d239 = floor_spacer_size"
equation "d240 = floor_spacer_size"
equation "d241 = floor_spacer_size"
equation "d242 = floor_spacer_size"
equation "d243 = floor_spacer_size"
equation "d244 = floor_spacer_size / 2"
equation "d245 = floor_spacer_size"
equation "d246 = floor_spacer_size / 2"
equation "d247 = floor_spacer_size"
equation "d248 = floor_spacer_size"
equation "d249 = floor_spacer_size"
equation "d250 = floor_spacer_size"
equation "floor_z_offset = batt_height / 2 - height"
equation "d252 = floor_z_offset"
equation "d255 = floor_fix_fillet"
equation "floor_fix_fillet = elem_fix_fillet"
equation "floor_fix_fillet_add = 5 mm"
equation "d259 = floor_fix_fillet_add"
equation "d260 = height + elem_fix_spacer_height"
equation "d261 = elem_fix_screw_hole_diam"
equation "d263 = height + elem_fix_spacer_height"
equation "d264 = elem_fix_screw_hole_diam"
equation "d266 = height + elem_fix_spacer_height"
equation "d267 = elem_fix_screw_hole_diam"
equation "d269 = height + elem_fix_spacer_height"
equation "d270 = elem_fix_screw_hole_diam"
equation "d272 = height + elem_fix_spacer_height"
equation "d273 = elem_fix_screw_hole_diam"
equation "d275 = height + elem_fix_spacer_height"
equation "d276 = elem_fix_screw_hole_diam"
equation "d278 = height + elem_fix_spacer_height"
equation "d279 = elem_fix_screw_hole_diam"
equation "d281 = height + elem_fix_spacer_height"
equation "d282 = elem_fix_screw_hole_diam"
equation "floor_cut_width = ( ( batt_width + batt_wall * 2 ) / 2 - ( bms_width + bms_wall * 2 ) / 2 ) + width - ( batt_wall * 2 + batt_width )"
equation "d285 = width"
equation "d286 = length - ( batt_length + batt_wall * 2 )"
equation "d287 = floor_cut_width"
equation "d288 = floor_cut_length"
equation "d289 = height"
equation "d291 = floor_spacer_size"
equation "d292 = floor_spacer_size"
equation "d293 = floor_spacer_size"
equation "d294 = floor_spacer_size"
equation "d295 = floor_spacer_size"
equation "d296 = floor_spacer_size"
equation "d297 = floor_spacer_size"
equation "d298 = floor_spacer_size"
equation "d299 = floor_spacer_size"
equation "d300 = floor_spacer_size"
equation "d301 = floor_spacer_size"
equation "d302 = bms_length + bms_wall * 2"
equation "d303 = floor_spacer_size"
equation "d304 = floor_spacer_size / 2"
equation "d305 = floor_spacer_size"
equation "d306 = floor_spacer_size / 2"
equation "d307 = floor_spacer_size"
equation "d308 = floor_spacer_size"
equation "floor_fix_screw_ext_hole_diam = 3 mm + slack_print"
equation "d310 = floor_fix_screw_ext_hole_diam"
equation "d311 = floor_fix_screw_ext_hole_diam"
equation "d312 = floor_fix_screw_ext_hole_diam"
equation "d313 = floor_fix_screw_ext_hole_diam"
equation "d314 = floor_fix_screw_ext_hole_diam"
equation "d315 = floor_fix_screw_ext_hole_diam"
equation "d316 = floor_fix_screw_ext_hole_diam"
equation "d317 = floor_fix_screw_ext_hole_diam"
equation "d326 = bms_width + bms_wall * 2"
equation "d327 = bms_wall"
equation "d328 = bms_thick + bms_wall * 2"
equation "d332 = -bms_wall"
equation "d335 = elem_fix_screw_hole_diam"
equation "d338 = elem_fix_screw_hole_diam"
equation "bms_fix_screw_ext_hole_diam = floor_fix_screw_ext_hole_diam - 0.5 mm"
equation "d341 = bms_fix_screw_ext_hole_diam"
equation "d344 = bms_fix_screw_ext_hole_diam"
equation "slack_print = 0.5 mm"
equation "d348 = -slack_print"
equation "d350 = -slack_print"
equation "d352 = -slack_print"
equation "d354 = -slack_print"
equation "d356 = -slack_print"
equation "d358 = -slack_print"
equation "d360 = -slack_print"
equation "d362 = -slack_print"
equation "d364 = -slack_print"
equation "d370 = -batt_wall - slack_print"
equation "d371 = -slack_print"
equation "batt_cover_height = batt_wall * 3"
equation "d373 = -batt_cover_height"
equation "d375 = batt_wall"
equation "d377 = batt_wall * 2"
equation "d378 = batt_wall"
equation "d379 = batt_wall"
equation "d380 = batt_wall"
equation "d381 = batt_wall * 2"
equation "d382 = batt_wall"
equation "d383 = batt_wall"
equation "d384 = batt_wall"
equation "d385 = elem_fix_screw_hole_diam"
equation "d386 = elem_fix_screw_hole_diam"
equation "d389 = batt_length + batt_wall * 2"
equation "d390 = batt_wall"
equation "d391 = batt_wall / 2"
equation "d392 = batt_wall"
equation "d393 = batt_wall / 2"
equation "d394 = batt_wall"
equation "d395 = elem_fix_screw_hole_diam"
equation "batt_cover_fix_screw_ext_hole_diam = floor_fix_screw_ext_hole_diam"
equation "d399 = batt_cover_fix_screw_ext_hole_diam"
equation "d400 = batt_cover_fix_screw_ext_hole_diam"
equation "d401 = batt_cover_fix_screw_ext_hole_diam"
equation "d406 = batt_wall"
equation "d407 = batt_wall + slack_print"
equation "d408 = batt_wall + slack_print"
equation "d409 = batt_wall"
equation "d410 = batt_wall"
equation "arduino_length = 57 mm"
equation "arduino_width = 113 mm"
equation "d420 = arduino_length"
equation "d421 = arduino_width"
equation "d428 = elem_fix_spacer_diam"
equation "d429 = elem_fix_spacer_diam"
equation "d430 = arduino_length"
equation "d436 = elem_fix_spacer_height"
equation "d443 = elem_fix_screw_hole_diam"
equation "d446 = elem_fix_screw_hole_diam"
equation "d449 = elem_fix_screw_hole_diam"
equation "d452 = elem_fix_screw_hole_diam"
equation "d455 = elem_fix_fillet"
equation "elem_fix_head_diam = 6.5 mm"
equation "elem_fix_head_height = 2.5 mm"
equation "d466 = -elem_fix_head_height"
equation "d468 = elem_fix_head_diam"
equation "d469 = elem_fix_head_diam"
equation "d470 = elem_fix_head_diam"
equation "d471 = elem_fix_head_diam"
equation "d472 = -elem_fix_head_height"
equation "d474 = elem_fix_head_diam"
equation "d475 = -elem_fix_head_height"
equation "d477 = elem_fix_head_diam"
equation "d478 = elem_fix_head_diam"
equation "d479 = elem_fix_head_diam"
equation "d480 = elem_fix_head_diam"
equation "d481 = elem_fix_head_diam"
equation "d482 = elem_fix_head_diam"
equation "d483 = elem_fix_head_diam"
equation "d484 = elem_fix_head_diam"
equation "d485 = elem_fix_head_diam"
equation "d486 = elem_fix_head_diam"
equation "d487 = elem_fix_head_diam"
equation "d488 = elem_fix_head_diam"
equation "d489 = elem_fix_head_diam"
equation "d490 = -elem_fix_head_height"
equation "d493 = elem_fix_fillet"
equation "d495 = elem_fix_fillet"
named bodies: "baseplate", "floor", "bms_fixate", "batt_cover"
